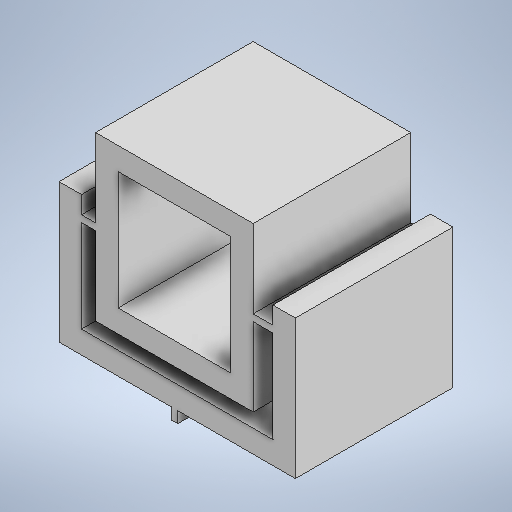
# Autodesk Inventor part: Pan-tilt _draw
Saved by Autodesk Inventor 2025 (Build 290162000, 162)
## iProperties
Created: 2024-04-08
Part Number: Pan-tilt _draw
Material: Generic
Document SubType Name: Modeling
Designer: Rikke
Density: 1 g/cm^3
Appearance: Default
Author: Rikke
Autodesk Inventor part; units mm, degrees
ref_plane "YZ Plane" through (0, 0, 0) normal (1, 0, 0) x (0, 1, 0)
ref_plane "XZ Plane" through (0, 0, 0) normal (0, 1, 0) x (-1, 0, 0)
ref_plane "XY Plane" through (0, 0, 0) normal (0, 0, 1) x (1, 0, 0)
sketch "Sketch1" plane through (0, 0, 0) normal (0, 0, 1) x (1, 0, 0)
  point P0 (0, 0)
sketch "Sketch2" plane through (0, 0, 0) normal (0, 0, 1) x (1, 0, 0)
  line L0 (-140, 105) -> (-140, -105)
  line L1 (-140, -105) -> (-100, -105)
  line L2 (-100, -105) -> (-100, 105)
  line L3 (-140, -105) -> (-140, -145)
  line L4 (-140, -145) -> (140, -145)
  line L5 (140, -145) -> (140, -105)
  line L6 (140, -105) -> (-140, -105)
  line L7 (140, -105) -> (140, 105)
  line L8 (100, 105) -> (100, -105)
  line L9 (140, 145) -> (-140, 145)
  line L10 (-140, 145) -> (-140, 105)
  line L11 (-140, 145) -> (-140, 139.6752)
  line L12 (-168.1795, -170) -> (215, -170)
  line L13 (215, -170) -> (215, -210)
  line L14 (215, -210) -> (-205, -210)
  line L15 (-205, -210) -> (-205, -170)
  line L16 (-205, -170) -> (215, -170)
  line L17 (-205, -170) -> (-165, -170)
  line L18 (-205, -210) -> (29.9617, -210)
  line L19 (29.9617, -210) -> (6, -210)
  line L20 (6, -210) -> (6, -230)
  line L21 (-6, -230) -> (-6, -210)
  line L22 (0, 174.1537) -> (0, -275.8463) construction
  line L23 (-230.7435, 0) -> (272.144, 0) construction
  line L24 (-6, -230) -> (6, -230)
  line L25 (140, 6) -> (175, 6)
  line L26 (140, -6) -> (175, -6)
  line L27 (215, -170) -> (175, -170)
  line L28 (175, -170) -> (175, 37)
  line L29 (175, 37) -> (215, 37)
  line L30 (215, 37) -> (215, -170)
  line L31 (-205, -170) -> (-165, -170)
  line L32 (-165, -170) -> (-165, 37)
  line L33 (-165, 37) -> (-205, 37)
  line L34 (-205, 37) -> (-205, -170)
  line L35 (-165, 6) -> (-140, 6)
  line L36 (-140, -6) -> (-165, -6)
  line L37 (140, 145) -> (140, 105)
  line L38 (-140, 105) -> (140, 105)
  point P0 (0, 0)
  dimension "d18" = 40
  dimension "d25" = 40
  dimension "d33" = 290
  dimension "d81" = 40
  dimension "d83" = 40
  dimension "d84" = 40
  dimension "d125" = 6
  dimension "d126" = 12
  dimension "d127" = 20
  dimension "d129" = 35
  dimension "d130" = 40
  dimension "d131" = 12
  dimension "d132" = 6
  dimension "d133" = 25
  dimension "d134" = 12
  dimension "d135" = 6
  dimension "d136" = 40
  dimension "d137" = 207
  dimension "d138" = 207
  dimension "d140" = 40
  dimension "d141" = 40
  dimension "d142" = 280
  dimension "d143" = 280
  dimension "d144" = 140
  dimension "d145" = 25
  dimension "d146" = 105
  constraints: 78 end point, 18 point on line, 16 perpendicular, 7 horizontal, 6 vertical, 4 parallel, 1 collinear
  measures "d18" distance of L0.end L1.end
  measures "d25" distance of L0.end L3.end
  measures "d33" distance of L4.end L9.start
  measures "d81" distance of L12.end L13.end
  measures "d83" distance of L14.end L15.end
  measures "d84" distance of L15.end L17.end
  measures "d125" distance between parallel lines of L22 L21
  measures "d126" distance between parallel lines of L21 L20
  measures "d127" distance between parallel lines of L14 L24
  measures "d129" distance of L25.start L25.end
  measures "d130" distance of L28.end L29.end
  measures "d131" distance between parallel lines of L26 L25
  measures "d132" distance between parallel lines of L23 L25
  measures "d133" distance between parallel lines of L0 L32
  measures "d134" distance between parallel lines of L36 L35
  measures "d135" distance between parallel lines of L23 L35
  measures "d136" distance of L32.end L33.end
  measures "d137" distance between parallel lines of L12 L33
  measures "d138" distance of L29.end L12.end
  measures "d140" distance of L9.start L7.end
  measures "d141" distance between parallel lines of L7 L8
  measures "d142" distance of L9.start L9.end
  measures "d143" distance of L3.end L4.end
  measures "d144" distance from line of L7 point (0, 0)
  measures "d145" distance between parallel lines of L12 L4
  measures "d146" distance from line of point (0, 0) L6
extrude "Extrusion1" add sketch "Sketch2" along normal blind 280 contours L38 L2 L1 L0 | L10 L9 L37 L38 | L0 L36 L32 L35 | L32 L12 L16 L34 L33 | L6 L5 L4 L3 L1 | L38 L7 L6 L8 | L12 L13 L14 L15 L16 | L25 L28 L26 L7 | L28 L29 L30 L12 | L14 L20 L24 L21
body "Solid1"
